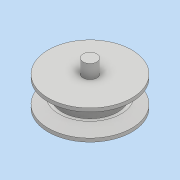
# Autodesk Inventor part: Ròng rọc 48mm
Saved by Autodesk Inventor 2018 (Build 220112000, 112)
## iProperties
Created: 2020-08-11
Part Number: Ròng rọc 48mm
Material: Generic
Document SubType Name: Modeling
Designer: ASUS
Density: 1 g/cm^3
Appearance: Default
Author: ASUS
Autodesk Inventor part; units mm, degrees
ref_plane "YZ Plane" through (0, 0, 0) normal (1, 0, 0) x (0, 1, 0)
ref_plane "XZ Plane" through (0, 0, 0) normal (0, 1, 0) x (-1, 0, 0)
ref_plane "XY Plane" through (0, 0, 0) normal (0, 0, 1) x (1, 0, 0)
sketch "Sketch1" plane through (0, 0, 0) normal (0, 1, 0) x (-1, 0, 0)
  line L0 (0, 0) -> (24, 0)
  line L1 (24, -17) -> (0, -17)
  line L2 (0, -17) -> (0, 0)
  line L3 (24, -2) -> (14, -2)
  line L4 (14, -2) -> (14, -15)
  line L5 (14, -15) -> (24, -15)
  line L6 (24, -2) -> (17.8462, -6)
  line L7 (24, -15) -> (17.8462, -11)
  line L8 (14, -6) -> (17.8462, -6)
  line L9 (17.8462, -11) -> (14, -11)
  line L10 (24, 0) -> (24, -2)
  line L11 (24, -15) -> (24, -17)
  line L12 (16, -6) -> (16, -11)
  dimension "d0" = 24
  dimension "d1" = 17
  dimension "d2" = 2
  dimension "d3" = 2
  dimension "d4" = 10
  dimension "d5" = 4
  dimension "d6" = 4
  dimension "d7" = 2
  constraints: 26 end point, 5 perpendicular, 4 parallel, 4 point on line, 3 horizontal
  measures "d0" distance of L1.start L1.end
  measures "d1" distance of L0.end L1.start
  measures "d2" distance between parallel lines of L0 L3
  measures "d3" distance between parallel lines of L1 L5
  measures "d4" distance of L4.end L5.end
  measures "d5" distance between parallel lines of L3 L8
  measures "d6" distance between parallel lines of L5 L9
  measures "d7" distance between parallel lines of L4 L12
revolve "Revolution1" add sketch "Sketch1" angle 360 about axis through (0, 0, -17) along (0, 0, 1)
sketch "Sketch2" plane through (0, 0, 0) normal (0, 0, 1) x (1, 0, 0)
  circle A0 centre (0, 0) radius 4
  dimension "d9" = 8
  constraints: 1 centre point, 1 coincident
  measures "d9" diameter of A0
extrude "Extrusion1" add sketch "Sketch2" against normal blind 24 and the other way blind 8
body "Solid1"
